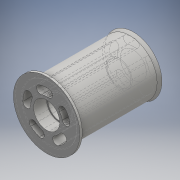
# Autodesk Inventor part: spooler big
Saved by Autodesk Inventor 2016 (Build 200138000, 138)
## iProperties
Created: 2016-02-14
Part Number: spooler big
Material: Generic
Document SubType Name: Modeling
Designer: Erwin
Density: 1 g/cm^3
Appearance: Default
Author: Erwin
Autodesk Inventor part; units mm, degrees
ref_plane "YZ Plane" through (0, 0, 0) normal (1, 0, 0) x (0, 1, 0)
ref_plane "XZ Plane" through (0, 0, 0) normal (0, 1, 0) x (-1, 0, 0)
ref_plane "XY Plane" through (0, 0, 0) normal (0, 0, 1) x (1, 0, 0)
sketch "Sketch1" plane through (0, 0, 0) normal (0, 1, 0) x (-1, 0, 0)
  circle A0 centre (0, 0) radius 11.05
  circle A1 centre (0, 0) radius 28
  dimension "d0" = 22.1
  dimension "d1" = 56
  constraints: 2 centre point, 2 coincident
  measures "d0" diameter of A0
  measures "d1" diameter of A1
extrude "Extrusion1" add sketch "Sketch1" along normal blind 2
sketch "Sketch2" plane through (0, 2, 0) normal (0, 1, 0) x (1, 0, 0)
  circle A0 centre (0, 0) radius 23
  dimension "d4" = 46
  constraints: 1 centre point, 1 coincident
  measures "d4" diameter of A0
extrude "Extrusion2" add sketch "Sketch2" along normal blind 68
sketch "Sketch3" plane through (0, 70, 0) normal (0, 1, 0) x (1, 0, 0)
  circle A0 centre (0, 0) radius 23 projected
extrude "Extrusion3" add sketch "Sketch3" along normal blind 3 draft 20
sketch "Sketch4" plane through (0, 2, 0) normal (0, -1, 0) x (1, 0, 0)
  circle A0 centre (0, 0) radius 11.05 projected
extrude "Extrusion4" cut sketch "Sketch4" against normal blind 9
sketch "Sketch5" plane through (0, 11, 0) normal (0, -1, 0) x (1, 0, 0)
  circle A0 centre (0, 0) radius 10
  dimension "d11" = 20
  constraints: 1 centre point, 1 coincident
  measures "d11" diameter of A0
extrude "Extrusion5" cut sketch "Sketch5" against normal up to next
sketch "Sketch6" plane through (0, 73, 0) normal (0, 1, 0) x (1, 0, 0)
  circle A0 centre (0, 0) radius 11.05
  dimension "d14" = 22.1
  constraints: 1 centre point, 1 coincident
  measures "d14" diameter of A0
extrude "Extrusion6" cut sketch "Sketch6" against normal blind 12
sketch "Sketch7" plane through (0, 0, 0) normal (0, -1, 0) x (1, 0, 0)
  circle A0 centre (0, 0) radius 11.05 projected
  circle A1 centre (0, 0) radius 28 projected
  line L0 (0, 0) -> (43.5603, 0) construction
  line L1 (-10.3416, 8.6776) -> (-15.3209, 12.8558) construction
  arc A2 (-15.3019, 6.8128) -> (-16.75, 0) centre (0, 0) ccw construction
  arc A3 (-18.2709, 8.1347) -> (-20, 0) centre (0, 0) ccw
  arc A4 (-12.3329, 5.4909) -> (-13.5, 0) centre (0, 0) ccw
  arc A5 (-12.3329, 5.4909) -> (-18.2709, 8.1347) centre (-15.3019, 6.8128) ccw
  arc A6 (-20, 0) -> (-13.5, 0) centre (-16.75, 0) ccw
  arc A7 (-9.0333, -10.0325) -> (-13.3826, -14.8629) centre (-11.2079, -12.4477) ccw
  arc A8 (-6.1803, -19.0211) -> (-4.1717, -12.8393) centre (-5.176, -15.9302) ccw
  arc A9 (6.75, -11.6913) -> (10, -17.3205) centre (8.375, -14.5059) ccw
  arc A10 (16.1803, -11.7557) -> (10.9217, -7.9351) centre (13.551, -9.8454) ccw
  arc A11 (13.205, 2.8068) -> (19.563, 4.1582) centre (16.384, 3.4825) ccw
  arc A12 (16.1803, 11.7557) -> (10.9217, 7.9351) centre (13.551, 9.8454) ccw
  arc A13 (1.4111, 13.426) -> (2.0906, 19.8904) centre (1.7509, 16.6582) ccw
  arc A14 (-6.1803, 19.0211) -> (-4.1717, 12.8393) centre (-5.176, 15.9302) ccw
  arc A15 (-12.3329, 5.4909) -> (-13.5, 0) centre (0, 0) ccw
  arc A16 (-18.2709, 8.1347) -> (-20, 0) centre (0, 0) ccw
  arc A17 (-13.3826, -14.8629) -> (-6.1803, -19.0211) centre (0, 0) ccw
  arc A18 (-9.0333, -10.0325) -> (-4.1717, -12.8393) centre (0, 0) ccw
  arc A19 (10, -17.3205) -> (16.1803, -11.7557) centre (0, 0) ccw
  arc A20 (6.75, -11.6913) -> (10.9217, -7.9351) centre (0, 0) ccw
  arc A21 (13.205, 2.8068) -> (10.9217, 7.9351) centre (0, 0) ccw
  arc A22 (1.4111, 13.426) -> (-4.1717, 12.8393) centre (0, 0) ccw
  arc A23 (19.563, 4.1582) -> (16.1803, 11.7557) centre (0, 0) ccw
  arc A24 (2.0906, 19.8904) -> (-6.1803, 19.0211) centre (0, 0) ccw
  point P0 (-12.8312, 10.7667)
  point P1 (-14.2048, 8.8761)
  point P2 (-16.1011, 4.6169)
  point P3 (-16.587, 2.3311)
  dimension "d22" = 40
  dimension "d26" = 360
  constraints: 47 point on circle, 23 centre point, 4 end point, 4 tangent, 2 coincident, 1 horizontal, 1 midpoint, 47 other
extrude "Extrusion7" cut sketch "Sketch7" against normal up to next contours A5 A4 A6 A3 | A18 A8 A17 A7 | A20 A10 A19 A9 | A21 A12 A23 A11 | A22 A14 A24 A13
fillet "Fillet1" radius 0.5 1 edges at (-23, 2, 0)
body "Solid1"
